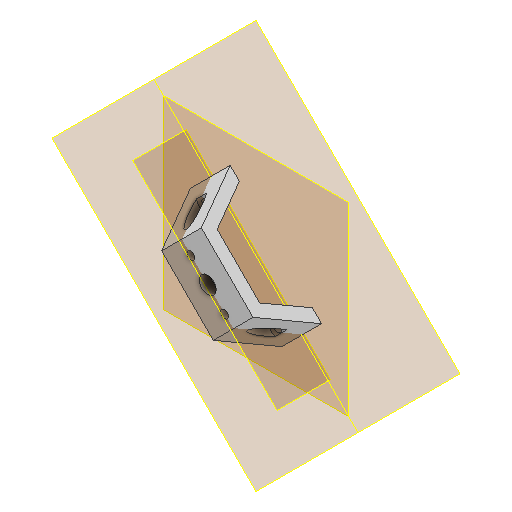
# Autodesk Inventor part: Anglerfish_Lightplate_Tislinkbridge
Saved by Autodesk Inventor 2022 (Build 260153000, 153)
## iProperties
Created: 2022-08-14
Part Number: Anglerfish_Lightplate_Tislinkbridge
Material: Generic
Document SubType Name: Modeling
Designer: diederichbenedict
Density: 1 g/cm^3
Appearance: Default
Author: diederichbenedict
Autodesk Inventor part; units mm, degrees
ref_plane "YZ Plane" through (0, 0, 0) normal (1, 0, 0) x (0, 1, 0)
ref_plane "XZ Plane" through (0, 0, 0) normal (0, 1, 0) x (-1, 0, 0)
ref_plane "Work Plane1" through (0, 0, 0) normal (0, 0, 1) x (1, 0, 0)
ref_plane "Work Plane2" through (0, 0, 0) normal (0, 0, 1) x (1, 0, 0)
ref_plane "Work Plane3" through (18.3844, -18.3844, 0) normal (0.7071, 0.7071, 0) x (-0.7071, 0.7071, 0)
sketch "Sketch2" plane through (18.3844, -18.3844, 0) normal (0.7071, 0.7071, 0) x (-0.7071, 0.7071, 0)
  line L0 (2.9994, 0) -> (12.9994, 17.3205)
  line L1 (-4.0006, 0) -> (15.9994, 0) construction
  line L2 (48.9994, 0) -> (38.9994, 17.3205)
  line L3 (56.0448, 0) -> (76.0448, 0) construction
  line L4 (38.9994, 17.3205) -> (12.9994, 17.3205)
  line L5 (7.6182, 0) -> (15.3088, 13.3205)
  line L6 (15.3088, 13.3205) -> (36.69, 13.3205)
  line L7 (36.69, 13.3205) -> (44.3806, 0)
  line L8 (-17.6765, -6) -> (-19.9184, -71) projected
  line L9 (53.3865, -6) -> (55.409, -71) projected
  line L10 (20.5601, 2) -> (20.5601, 10)
  line L11 (33.5601, 2) -> (33.5601, 10)
  line L12 (48, 0) -> (-12, 0) projected
  line L13 (44.3806, 0) -> (48.9994, 0)
  line L14 (2.9994, 0) -> (7.6182, 0)
  line L15 (-4.0006, -9.8008) -> (-4.0006, -30.1937)
  line L16 (55.9994, -9.8008) -> (55.9994, -30.1937)
  point P0 (25.9994, 0)
  dimension "d1" = 20
  dimension "d2" = 60
  dimension "d3" = 120
  dimension "d5" = 4
  dimension "d6" = 4
  dimension "d7" = 4
  dimension "d24" = 7
  dimension "d25" = 7
  constraints: 28 end point, 5 horizontal, 4 vertical, 2 equal length, 2 parallel, 2 point on line, 13 other
  measures "d1" distance of L0.start L0.end
  measures "d2" angle of L1 L0
  measures "d3" angle of L3 L2
  measures "d5" distance between parallel lines of L5 L0
  measures "d6" distance between parallel lines of L2 L7
  measures "d7" distance between parallel lines of L4 L6
  measures "d24" distance from line of L0.start L15
  measures "d25" distance from line of L16 L2.start
extrude "Extrusion1" add sketch "Sketch2" along normal mid plane 20 contours L0 L4 L2 L13 L12 L7 L6 L5
sketch "Sketch3" plane through (16.2635, -2.1213, 17.3205) normal (0, 0, 1) x (0.7071, 0.7071, 0)
  circle A0 centre (-9.3718, 30.7817) radius 1.4 projected
  circle A1 centre (-10.6281, -5.1964) radius 1.4 projected
  line L0 (-20, -5.3812) -> (0, -5.3812) projected
  point P0 (-9.968, 30.7817)
  point P1 (-10, -5.3812)
  constraints: 1 midpoint
hole "Hole1" at (-12.5509, 12.5962, 17.3205) at (12.9975, -12.9975, 17.3205) direction (0, 0, -1) diameter 2.8 end through all counterbore diameter 6.5 counterbore depth 12
sketch "Sketch4" plane through (16.2635, -2.1213, 17.3205) normal (0, 0, 1) x (0.7071, 0.7071, 0)
  circle A0 centre (-10.0015, 21.2913) radius 1.9 projected
  line L0 (0, 26) -> (0, 0) projected
  line L1 (-20, 0) -> (-20, 26) projected
  circle A1 centre (-10.0015, 4.2912) radius 1.9 projected
  circle A2 centre (-10.0015, 12.7912) radius 3 projected
  circle A3 centre (-10.0015, 21.2913) radius 1.4
  circle A4 centre (-10.0015, 4.2912) radius 1.9
  circle A5 centre (-10.0015, 4.2912) radius 1.4
  line L2 (-20, 26) -> (0, 26) projected
  line L3 (-20, 0) -> (0, 0) projected
  point P0 (-10, 13)
  dimension "d17" = 2.8
  dimension "d18" = 2.8
  constraints: 3 centre point, 3 coincident, 1 concentric
  measures "d17" diameter of A3
  measures "d18" diameter of A5
extrude "Extrusion2" cut sketch "Sketch4" against normal blind 20 contours A2 | A3 | A5
ref_plane "Arbeitsebene4" through (18.3844, -18.3844, 0) normal (0.7071, 0.7071, 0) x (0, 0, 1)
body "Solid1"
